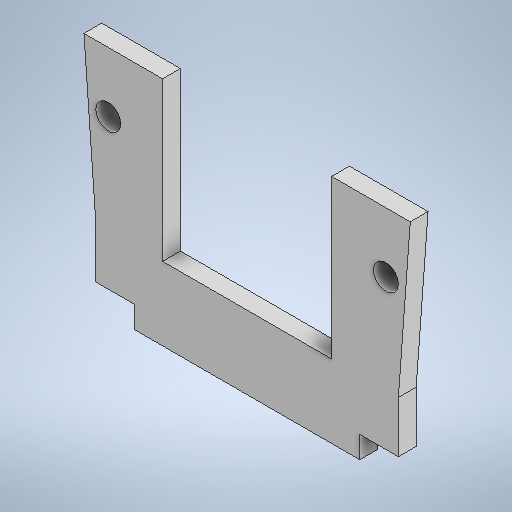
# Autodesk Inventor part: A
Saved by Autodesk Inventor 2025.3 (Build 293356030, 356C)
## iProperties
Created: 2025-07-09
Part Number: A
Material: Generic
Document SubType Name: Modeling
Designer: jv
Density: 1 g/cm^3
Appearance: Default
Author: jv
Autodesk Inventor part; units mm, degrees
ref_plane "YZ Plane" through (0, 0, 0) normal (1, 0, 0) x (0, 1, 0)
ref_plane "XZ Plane" through (0, 0, 0) normal (0, 1, 0) x (-1, 0, 0)
ref_plane "XY Plane" through (0, 0, 0) normal (0, 0, 1) x (1, 0, 0)
sketch "Sketch1" plane through (0, 0, 0) normal (0, 0, 1) x (1, 0, 0)
  line L0 (-27.5, 38.9876) -> (27.5, 38.9876)
  line L1 (27.5, 38.9876) -> (27.5, 0)
  line L2 (27.5, 0) -> (-27.5, 0)
  line L3 (-27.5, 0) -> (-27.5, 38.9876)
  line L4 (-19, 0) -> (19, 0)
  line L5 (19, 0) -> (19, 3.7)
  line L6 (19, 3.7) -> (-19, 3.7)
  line L7 (-19, 3.7) -> (-19, 0)
  line L8 (-25.5, 12.34) -> (25.5, 12.34)
  line L9 (25.5, 12.34) -> (25.5, 3.7)
  line L10 (25.5, 3.7) -> (-25.5, 3.7)
  line L11 (-25.5, 3.7) -> (-25.5, 12.34)
  line L12 (27.5, 38.9876) -> (25.5, 12.34)
  line L13 (-25.5, 12.34) -> (-27.5, 38.9876)
  circle A0 centre (23.4, 28.8876) radius 2.1
  line L14 (0, 12.34) -> (0, 0)
  circle A1 centre (-23.4, 28.8876) radius 2.1
  line L15 (-14.25, 38.9876) -> (14.25, 38.9876)
  line L16 (14.25, 38.9876) -> (14.25, 12.34)
  line L17 (14.25, 12.34) -> (-14.25, 12.34)
  line L18 (-14.25, 12.34) -> (-14.25, 38.9876)
  point P0 (0, 6.1823)
  point P1 (0, 3.7)
  point P2 (0, 38.9876)
  point P3 (19, 0)
  dimension "d0" = 55
  dimension "d1" = 3.7
  dimension "d2" = 8.64
  dimension "d3" = 38
  dimension "d4" = 51
  dimension "d5" = 4.2
  dimension "d6" = 10.1
  dimension "d8" = 4.1
  dimension "d9" = 28.5
  constraints: 38 end point, 8 parallel, 7 midpoint, 4 horizontal, 4 perpendicular, 3 point on line, 2 centre point, 1 coincident, 1 symmetric about line, 1 vertical, 1 vertical alignment, 1 other
  measures "d0" distance of L0.start L0.end
  measures "d1" distance of L4.end L5.end
  measures "d2" distance of L8.end L9.end
  measures "d3" distance of L5.end L6.end
  measures "d4" distance of L8.start L8.end
  measures "d5" diameter of A0
  measures "d6" distance from line of L0 A0.centre
  measures "d8" distance from line of L1 A0.centre
  measures "d9" distance between parallel lines of L16 L18
extrude "Extrusion1" add sketch "Sketch1" along normal mid plane 3 contours L0 L18 L8 L13 | L8 L14 L6 L10 L11 | L0 L12 L8 L16 | L7 L6 L14 L2 | L8 L9 L10 L6 L14 | L14 L6 L5 L2
body "Solid1"
